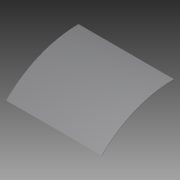
# Autodesk Inventor part: Back
Saved by Autodesk Inventor 2013 (Build 170138000, 138)
## iProperties
Created: 2013-01-27
Part Number: Back
Material: Polycarbonate, Clear
Document SubType Name: Modeling
Designer: Andrew Toennies
Density: 1.2 g/cm^3
Mass: 127.858 g
Surface Area: 1358.85 cm^2
Volume: 106.548 cm^3
Author: Andrew Toennies
Autodesk Inventor part; units mm, degrees
ref_plane "YZ Plane" through (0, 0, 0) normal (1, 0, 0) x (0, 1, 0)
ref_plane "XZ Plane" through (0, 0, 0) normal (0, 1, 0) x (-1, 0, 0)
ref_plane "XY Plane" through (0, 0, 0) normal (0, 0, 1) x (1, 0, 0)
sketch "Sketch1" plane through (0, 0, 0) normal (1, 0, 0) x (0, 1, 0)
  arc A0 (301.625, 0) -> (213.2811, 213.2811) centre (0, 0) ccw
  arc A1 (303.2125, 0) -> (214.4036, 214.4036) centre (0, 0) ccw
  line L0 (0, 0) -> (471.039, 0)
  line L1 (0, 0) -> (335.2588, 335.2588)
  dimension "d0" = 603.25
  dimension "d1" = 1.5875
  dimension "d2" = 45
  constraints: 4 end point, 4 point on circle, 4 point on line, 2 centre point, 2 coincident, 1 horizontal
  measures "d0" diameter of A0
  measures "d1" radial gap between concentric circles of A1 A0
  measures "d2" angle of L0 L1
extrude "Extrusion1" add sketch "Sketch1" along normal blind 282.575 contours A0 L1 A1 L0
body "Solid1"
